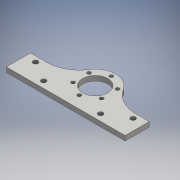
# Autodesk Inventor part: x axis nut support
Saved by Autodesk Inventor 2016 (Build 200138000, 138)
## iProperties
Created: 2017-06-27
Part Number: x axis nut support
Material: Generic
Document SubType Name: Modeling
Designer: M228544
Density: 1 g/cm^3
Appearance: Default
Author: M228544
Autodesk Inventor part; units mm, degrees
ref_plane "YZ Plane" through (0, 0, 0) normal (1, 0, 0) x (0, 1, 0)
ref_plane "XZ Plane" through (0, 0, 0) normal (0, 1, 0) x (-1, 0, 0)
ref_plane "XY Plane" through (0, 0, 0) normal (0, 0, 1) x (1, 0, 0)
sketch "Sketch1" plane through (0, 0, 0) normal (0, 0, 1) x (1, 0, 0)
  line L0 (-72.8091, 16.3486) -> (-72.8091, -13.2514) projected
  line L1 (-72.8091, -13.2514) -> (73.1909, -13.2514) projected
  line L2 (73.1909, -13.2514) -> (73.1909, 16.3486) projected
  line L3 (-72.8091, 16.3486) -> (-72.8091, 50.3486)
  line L4 (-72.8091, 50.3486) -> (73.1909, 50.3486)
  line L5 (73.1909, 50.3486) -> (73.1909, 16.3486)
  point P0 (0, 0)
  dimension "d0" = 34
  constraints: 6 end point, 1 collinear, 1 perpendicular, 1 vertical
  measures "d0" distance of L0.start L3.end
extrude "Extrusion1" add sketch "Sketch1" along normal blind 6
sketch "Sketch2" plane through (0, 0, 6) normal (0, 0, 1) x (1, 0, 0)
  circle A0 centre (35, -5.2514) radius 3
  circle A1 centre (60, 9.7486) radius 3
  line L0 (0, 0) -> (0, 8.3537) construction
  circle A2 centre (-35, -5.2514) radius 3
  circle A3 centre (-60, 9.7486) radius 3
  line L1 (-72.8091, -13.2514) -> (73.1909, -13.2514) projected
  dimension "d3" = 6
  dimension "d4" = 6
  dimension "d6" = 15
  dimension "d7" = 60
  dimension "d10" = 8
  dimension "d11" = 35
  constraints: 4 centre point, 2 end point, 2 symmetric about line, 1 vertical, 2 other
  measures "d3" diameter of A0
  measures "d4" diameter of A1
  measures "d6" vertical distance of A1.centre A0.centre
  measures "d7" horizontal distance of L0.start A1.centre
  measures "d10" distance from line of A0.centre L1
  measures "d11" horizontal distance of L0.start A0.centre
extrude "Extrusion2" cut sketch "Sketch2" against normal through all
sketch "Sketch3" plane through (0, 0, 6) normal (0, 0, 1) x (1, 0, 0)
  circle A0 centre (2.1259, 1.3506) radius 2.25
  circle A1 centre (-15.3355, 11.1025) radius 2.25
  circle A2 centre (-15.6209, 31.1004) radius 2.25
  circle A3 centre (1.5552, 41.3465) radius 2.25
  circle A4 centre (19.0166, 31.5947) radius 2.25
  circle A5 centre (19.302, 11.5967) radius 2.25
  circle A6 centre (1.8405, 21.3486) radius 15 construction
  circle A7 centre (1.8405, 21.3486) radius 15.5
  point P0 (0, 0)
extrude "Extrusion3" cut sketch "Sketch3" against normal through all
sketch "Sketch5" plane through (0, 0, 0) normal (0, 0, -1) x (-1, 0, 0)
  line L0 (-73.1909, 16.3486) -> (-40.1909, 16.3486) projected
  line L1 (42.9091, 16.3486) -> (72.8091, 16.3486) projected
  circle A0 centre (-1.8405, 21.3486) radius 25 construction
  line L2 (-40.1909, 16.3486) -> (-26.3354, 16.3486)
  line L3 (42.9091, 16.3486) -> (22.6544, 16.3486)
  arc A1 (22.6544, 16.3486) -> (-26.3354, 16.3486) centre (-1.8405, 21.3486) ccw
  line L4 (-73.1909, 50.3486) -> (72.8091, 50.3486) projected
  line L5 (-73.1909, 50.3486) -> (72.8091, 50.3486) projected
  line L6 (72.8091, 16.3486) -> (72.8091, 50.3486)
  line L7 (-73.1909, 50.3486) -> (-73.1909, 16.3486)
  line L8 (-73.1909, -13.2514) -> (-73.1909, 50.3486) projected
  point P0 (0, 0)
  constraints: 8 end point, 4 point on circle, 1 centre point, 1 coincident, 1 collinear, 1 horizontal, 1 perpendicular, 1 point on line
extrude "Extrusion4" cut sketch "Sketch5" against normal through all
fillet "Fillet2" radius 40 2 edges at (-22.6544, 16.3486, 3) (26.3354, 16.3486, 3)
body "Solid1"
